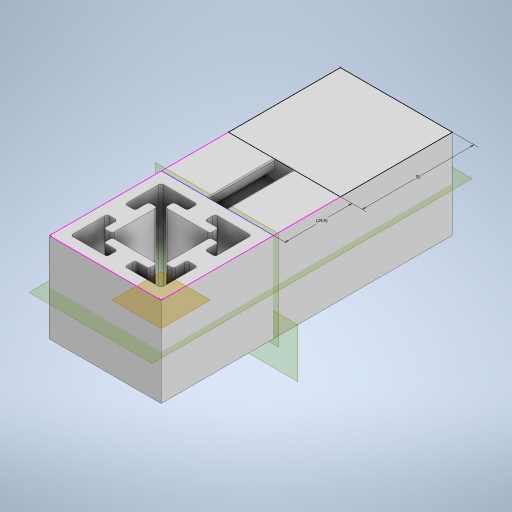
# Autodesk Inventor part: 임시저장
Saved by Autodesk Inventor 2023 (Build 270158000, 158)
## iProperties
Created: 2023-10-31
Part Number: 임시저장
Material: 일반
Document SubType Name: Modeling
Designer: rlatk
Density: 1 g/cm^3
Appearance: 기본값
Author: rlatk
Autodesk Inventor part; units mm, degrees
ref_plane "YZ Plane" through (0, 0, 0) normal (1, 0, 0) x (0, 1, 0)
ref_plane "XZ Plane" through (0, 0, 0) normal (0, 1, 0) x (-1, 0, 0)
ref_plane "XY Plane" through (0, 0, 0) normal (0, 0, 1) x (1, 0, 0)
sketch "스케치1" plane through (0, 0, 0) normal (0, 1, 0) x (-1, 0, 0)
  line L0 (0, 0) -> (50, 0)
  line L1 (50, 0) -> (50, -50)
  line L2 (50, -50) -> (0, -50)
  line L3 (0, -50) -> (0, 0)
  line L4 (45.2, -45.2) -> (4.8, -45.2)
  line L5 (4.8, -45.2) -> (4.8, -4.8)
  line L6 (4.8, -4.8) -> (45.2, -4.8)
  line L7 (45.2, -4.8) -> (45.2, -45.2)
  line L8 (28.95, -45.2) -> (21.05, -45.2)
  line L9 (21.05, -45.2) -> (21.05, -40.6)
  line L10 (21.05, -40.6) -> (28.95, -40.6)
  line L11 (28.95, -40.6) -> (28.95, -45.2)
  line L12 (35.05, -40.6) -> (14.95, -40.6)
  line L13 (14.95, -40.6) -> (14.95, -36.8)
  line L14 (14.95, -36.8) -> (35.05, -36.8)
  line L15 (35.05, -36.8) -> (35.05, -40.6)
  line L16 (45.2, -28.95) -> (40.6, -28.95)
  line L17 (40.6, -21.05) -> (45.2, -21.05)
  line L18 (40.6, -28.95) -> (40.6, -21.05)
  line L19 (40.6, -14.95) -> (40.6, -35.05)
  line L20 (36.8, -35.05) -> (36.8, -14.95)
  line L21 (36.8, -14.95) -> (40.6, -14.95)
  line L22 (40.6, -35.05) -> (36.8, -35.05)
  line L23 (45.2, -21.05) -> (45.2, -28.95)
  line L24 (28.95, -4.8) -> (28.95, -9.4)
  line L25 (21.05, -9.4) -> (21.05, -4.8)
  line L26 (28.95, -9.4) -> (21.05, -9.4)
  line L27 (14.95, -9.4) -> (35.05, -9.4)
  line L28 (35.05, -13.2) -> (14.95, -13.2)
  line L29 (14.95, -13.2) -> (14.95, -9.4)
  line L30 (35.05, -9.4) -> (35.05, -13.2)
  line L31 (21.05, -4.8) -> (28.95, -4.8)
  line L32 (4.8, -21.05) -> (9.4, -21.05)
  line L33 (9.4, -28.95) -> (4.8, -28.95)
  line L34 (9.4, -21.05) -> (9.4, -28.95)
  line L35 (9.4, -35.05) -> (9.4, -14.95)
  line L36 (13.2, -14.95) -> (13.2, -35.05)
  line L37 (13.2, -35.05) -> (9.4, -35.05)
  line L38 (9.4, -14.95) -> (13.2, -14.95)
  line L39 (4.8, -28.95) -> (4.8, -21.05)
  point P0 (25, -45.2)
  point P1 (25, -40.6)
  point P2 (25, -25)
  point P3 (21.05, -40.6)
  point P4 (40.6, -25)
  point P5 (45.2, -25)
  point P6 (25, -9.4)
  point P7 (25, -4.8)
  point P8 (9.4, -25)
  point P9 (4.8, -25)
  dimension "d0" = 50
  dimension "d1" = 50
  dimension "d2" = 40.4
  dimension "d3" = 40.4
  dimension "d4" = 4.8
  dimension "d5" = 4.8
  dimension "d6" = 7.9
  dimension "d7" = 4.6
  dimension "d8" = 20.1
  dimension "d9" = 3.8
  dimension "d43" = 360
  constraints: 80 end point, 8 parallel, 4 horizontal, 4 midpoint, 4 perpendicular, 73 other
  measures "d0" distance of L1.end L2.end
  measures "d1" distance of L0.end L1.end
  measures "d2" distance of L5.end L6.end
  measures "d3" distance of L4.end L5.end
  measures "d4" distance between parallel lines of L1 L7
  measures "d5" distance between parallel lines of L4 L2
  measures "d6" distance of L9.end L10.end
  measures "d7" distance of L8.end L9.end
  measures "d8" distance of L13.end L14.end
  measures "d9" distance of L12.end L13.end
ref_plane "작업 평면3" through (0, 0, -50) normal (0, 0, -1) x (-1, 0, 0)
sketch "스케치3" plane through (0, 0, -50) normal (0, 0, -1) x (-1, 0, 0)
  line L0 (50, 0) -> (50, 40) projected
  line L1 (0, 0) -> (0, 40) projected
  line L2 (50, 40) -> (0, 40)
  line L3 (0, 40) -> (0, 0)
  line L4 (0, 0) -> (50, 0)
  line L5 (50, 0) -> (50, 40)
  constraints: 8 end point, 2 parallel, 1 horizontal, 1 perpendicular
extrude "돌출2" add sketch "스케치3" along normal blind 80
ref_plane "작업 평면4" through (0, 40, 0) normal (0, 1, 0) x (1, 0, 0)
sketch "스케치4" plane through (0, 40, 0) normal (0, 1, 0) x (1, 0, 0)
  line L0 (-50, 1) -> (-50, 130) projected
  line L1 (0, 1) -> (0, 130) projected
  line L2 (-50, 130) -> (0, 130)
  line L3 (0, 130) -> (0, 80)
  line L4 (0, 80) -> (-50, 80)
  line L5 (-50, 80) -> (-50, 130)
  point P0 (0, 0)
  dimension "d19" = 50
  constraints: 8 end point, 2 parallel, 1 horizontal, 1 perpendicular, 1 point on line
  measures "d19" distance of L2.end L3.end
ref_plane "작업 평면5" through (0, 40, 0) normal (0, 1, 0) x (1, 0, 0)
sketch "스케치5" plane through (0, 40, 0) normal (0, 1, 0) x (1, 0, 0)
  arc A0 (-1, 0) -> (0, 1) centre (-1, 1) ccw projected
  line L0 (0, 1) -> (0, 130) projected
  line L1 (-50, 130) -> (0, 130) projected
  line L2 (-50, 1) -> (-50, 130) projected
  arc A1 (-50, 1) -> (-49, 0) centre (-49, 1) ccw projected
  line L3 (-49, 0) -> (-1, 0) projected
  line L4 (-50, 50.1) -> (0, 50.1)
  line L5 (0, 80) -> (-50, 80) projected
  point P0 (0, 0)
  dimension "d21" = 29.9
  constraints: 2 end point, 2 point on line, 1 perpendicular
  measures "d21" distance between parallel lines of L5 L4
ref_plane "작업 평면1" through (0, 0, -50) normal (0, 0, -1) x (-1, 0, 0)
sketch "스케치6" plane through (0, 0, -50) normal (0, 0, -1) x (-1, 0, 0)
  line L0 (20.85, 40) -> (29.15, 40)
  line L1 (29.15, 39.5) -> (29.15, 36.3)
  line L2 (29.15, 35.8) -> (20.85, 35.8)
  line L3 (20.85, 36.3) -> (20.85, 39.5)
  line L4 (50, 40) -> (0, 40) projected
  line L5 (19.05, 35.8) -> (20.35, 35.8)
  line L6 (35.25, 35.8) -> (35.25, 31.7)
  line L7 (35.25, 31.7) -> (14.75, 31.7)
  line L8 (14.75, 31.7) -> (14.75, 35.8)
  line L9 (14.75, 31.7) -> (35.25, 31.7)
  line L10 (35.25, 31.7) -> (35.25, 26.7)
  line L11 (35.25, 26.7) -> (14.75, 26.7)
  line L12 (14.75, 26.7) -> (14.75, 31.7)
  line L13 (14.75, 31.7) -> (19.75, 26.7)
  line L14 (14.75, 31.7) -> (21.8211, 31.7) construction
  line L15 (35.25, 31.7) -> (30.25, 26.7)
  line L16 (18.55, 36.3) -> (18.55, 37.2)
  line L17 (18.05, 37.7) -> (16.25, 37.7)
  line L18 (14.75, 36.2) -> (14.75, 35.8)
  line L19 (31.45, 36.3) -> (31.45, 37.2)
  line L20 (31.95, 37.7) -> (33.75, 37.7)
  line L21 (35.25, 36.2) -> (35.25, 35.8)
  arc A0 (16.25, 37.7) -> (14.75, 36.2) centre (16.25, 36.2) ccw
  arc A1 (35.25, 36.2) -> (33.75, 37.7) centre (33.75, 36.2) ccw
  line L22 (35.25, 35.8) -> (35.1957, 35.8)
  line L23 (32.3043, 35.8) -> (31.45, 35.8)
  arc A2 (18.55, 36.3) -> (19.05, 35.8) centre (19.05, 36.3) ccw
  arc A3 (18.55, 37.2) -> (18.05, 37.7) centre (18.05, 37.2) ccw
  arc A4 (20.35, 35.8) -> (20.85, 36.3) centre (20.35, 36.3) ccw
  line L24 (30.95, 35.8) -> (29.65, 35.8)
  arc A5 (29.15, 36.3) -> (29.65, 35.8) centre (29.65, 36.3) ccw
  arc A6 (31.95, 37.7) -> (31.45, 37.2) centre (31.95, 37.2) ccw
  arc A7 (30.95, 35.8) -> (31.45, 36.3) centre (30.95, 36.3) ccw
  line L25 (0, 40) -> (20.35, 40)
  arc A8 (20.85, 39.5) -> (20.35, 40) centre (20.35, 39.5) ccw
  line L26 (29.65, 40) -> (50, 40)
  arc A9 (29.65, 40) -> (29.15, 39.5) centre (29.65, 39.5) ccw
  line L27 (20.35, 40) -> (29.65, 40)
  line L28 (29.05, 40) -> (34.15, 40) projected
  point P0 (0, 0)
  point P1 (25, 40)
  point P2 (25, 35.8)
  point P3 (18.55, 37.7)
  point P4 (14.75, 37.7)
  point P5 (31.45, 37.7)
  point P6 (35.25, 37.7)
  point P7 (18.55, 35.8)
  dimension "d23" = 8.3
  dimension "d24" = 4.2
  dimension "d25" = 20.5
  dimension "d26" = 4.1
  dimension "d27" = 5
  dimension "d28" = 45
  dimension "d29" = 3.8
  dimension "d30" = 1.9
  dimension "d31" = 3.8
  dimension "d32" = 1.9
  dimension "d33" = 1.5
  dimension "d34" = 0.5
  dimension "d35" = 0.5
  dimension "d36" = 0.5
  dimension "d37" = 0.5
  constraints: 54 end point, 23 point on line, 22 point on circle, 20 tangent, 11 parallel, 10 centre point, 7 horizontal, 5 equal radius, 5 perpendicular, 3 midpoint, 2 collinear, 1 equal length
  measures "d23" distance of L2.start L2.end
  measures "d24" distance of L0.end L2.start
  measures "d25" distance of L6.end L7.end
  measures "d26" distance of L6.start L6.end
  measures "d27" distance of L9.end L10.end
  measures "d28" angle of L13 L14
  measures "d29" distance of point (14.75, 37.7) point (18.55, 37.7)
  measures "d30" distance of point (18.55, 35.8) point (18.55, 37.7)
  measures "d31" distance of point (31.45, 37.7) point (35.25, 37.7)
  measures "d32" distance of L23.end point (31.45, 37.7)
  measures "d33" radius of A0
  measures "d34" radius of A2
  measures "d35" radius of A5
  measures "d36" radius of A8
  measures "d37" radius of A9
extrude "돌출3" cut sketch "스케치6" along normal blind 30 contours L0 L4 A9 L1 A5 L24 A7 L19 A6 L20 A1 L21 L6 L7 L8 L18 A0 L17 A3 L16 A2 L5 A4 L3 A8
ref_plane "작업 평면2" through (0, 20, 0) normal (0, -1, 0) x (1, 0, 0)
mirror "미러1" about plane through (0, 20, 0) normal (0, -1, 0) of "돌출3"
extrude "돌출4" add sketch "스케치1" along normal blind 40 contours L0 L1 L2 L3 | L4 L9 L10 L11 | L16 L18 L17 L7 | L10 L12 L13 L14 L15 | L19 L22 L20 L21 L18 | L5 L32 L34 L33 | L24 L26 L25 L6 | L34 L35 L38 L36 L37 | L27 L30 L28 L29 L26
fillet "모깎기2" radius 1 8 edges at (-14.95, 20, -13.2) (-35.05, 20, -13.2) (-14.95, 20, -9.4) (-21.05, 20, -9.4) (-21.05, 20, -4.8) (-28.95, 20, -4.8) (-28.95, 20, -9.4) (-35.05, 20, -9.4)
fillet "모깎기3" radius 1 28 edges at (-13.2, 20, -14.95) (-9.4, 20, -14.95) (-4.8, 20, -21.05) (-9.4, 20, -21.05) (-9.4, 20, -28.95) (-4.8, 20, -28.95) (-9.4, 20, -35.05) (-13.2, 20, -35.05) (-36.8, 20, -14.95) (-40.6, 20, -14.95) (-36.8, 20, -35.05) (-40.6, 20, -35.05) (-40.6, 20, -28.95) (-45.2, 20, -28.95) (-40.6, 20, -21.05) (-45.2, 20, -21.05) (-35.05, 20, -36.8) (-14.95, 20, -36.8) (-14.95, 20, -40.6) (-21.05, 20, -40.6) (-21.05, 20, -45.2) (-28.95, 20, -45.2) (-28.95, 20, -40.6) (-35.05, 20, -40.6) (-4.8, 20, -4.8) (-45.2, 20, -4.8) (-4.8, 20, -45.2) (-45.2, 20, -45.2)
